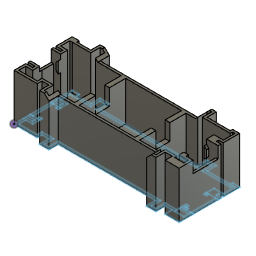
ICC Plug v2 v21 (Autodesk Fusion 360 design; units mm, degrees)
Autodesk Fusion 360 part; units mm, degrees
note: some values were not read from the file. Set by a fixed rule: which sketch regions a step uses.
sketch "Sketch1" plane through (0, 0, 0) normal (0, 1, 0) x (1, 0, 0)
  line L0 (3, 25) -> (0, 25)
  line L1 (0, 25) -> (0, 19)
  line L2 (0, 18) -> (3, 18)
  line L3 (3, 18) -> (3, 17)
  line L4 (3, 17) -> (0, 17)
  line L5 (0, 16) -> (0, 7)
  line L6 (0, 6) -> (3, 6)
  line L7 (3, 6) -> (3, 5)
  line L8 (3, 5) -> (0, 5)
  line L9 (0, 4) -> (0, 0)
  line L10 (0, 0) -> (10, 0)
  line L11 (10, 0) -> (10, 2)
  line L12 (10, 2) -> (13, 2)
  line L13 (13, 2) -> (13, -2)
  line L14 (13, -2) -> (17, -2)
  line L15 (17, -2) -> (17, 2)
  line L16 (17, 2) -> (59, 2)
  line L17 (59, 2) -> (59, -2)
  line L18 (59, -2) -> (63, -2)
  line L19 (63, -2) -> (63, 2)
  line L20 (63, 2) -> (66, 2)
  line L21 (66, 2) -> (66, -1.0002)
  line L22 (66, -1.0002) -> (72, -1.0002)
  line L23 (72, 24.9998) -> (69, 24.9998)
  line L24 (69, 24.9998) -> (69, 23.9998)
  line L25 (69, 23.9998) -> (59, 23.9998)
  line L26 (59, 23.9998) -> (59, 27.9998)
  line L27 (59, 27.9998) -> (55, 27.9998)
  line L28 (55, 27.9998) -> (55, 23.9998)
  line L29 (55, 23.9998) -> (13, 24)
  line L30 (13, 24) -> (13, 28)
  line L31 (13, 28) -> (9, 28)
  line L32 (9, 28) -> (9, 24)
  line L33 (9, 24) -> (3, 24)
  line L34 (3, 25) -> (3, 24)
  line L35 (72, -1.0002) -> (72, 4.9998)
  line L36 (72, 16.9998) -> (70, 16.9998)
  line L37 (70, 16.9998) -> (70, 17.9998)
  line L38 (70, 17.9998) -> (72, 17.9998)
  line L39 (72, 24.9998) -> (72, 18.9998)
  line L40 (72, 16.9998) -> (72, 15.7629)
  line L41 (72, 17.9998) -> (72, 18.9998)
  line L42 (0, 18) -> (0, 19)
  line L43 (0, 17) -> (0, 16)
  line L44 (0, 6) -> (0, 7)
  line L45 (0, 5) -> (0, 4)
  line L46 (12, 27) -> (10, 27)
  line L47 (10, 27) -> (10, 23)
  line L48 (10, 23) -> (2, 23)
  line L49 (1, 23) -> (1, 19)
  line L50 (1, 19) -> (4, 19)
  line L51 (4, 19) -> (4, 16)
  line L52 (4, 16) -> (1, 16)
  line L53 (1, 16) -> (1, 7)
  line L54 (1, 7) -> (4, 7)
  line L55 (4, 7) -> (4, 4)
  line L56 (4, 4) -> (1, 4)
  line L57 (1, 4) -> (1, 1)
  line L58 (1, 1) -> (9, 1)
  line L59 (9, 1) -> (9, 3)
  line L60 (9, 3) -> (14, 3)
  line L61 (14, 3) -> (14, -1)
  line L62 (14, -1) -> (16, -1)
  line L63 (16, -1) -> (16, 3)
  line L64 (16, 3) -> (60, 3)
  line L65 (60, 3) -> (60, -1)
  line L66 (60, -1) -> (62, -1)
  line L67 (62, -1) -> (62, 3)
  line L68 (62, 3) -> (67, 3)
  line L69 (67, 3) -> (67, 1.9998)
  line L70 (67, 1.9998) -> (71, 1.9998)
  line L71 (71, 1.9998) -> (71, 4.9998)
  line L72 (71, 15.7629) -> (67, 15.7629)
  line L73 (67, 15.7629) -> (67, 18.9998)
  line L74 (67, 18.9998) -> (71, 18.9998)
  line L75 (71, 23.9998) -> (71, 18.9998)
  line L76 (71, 23.9998) -> (70, 23.9998)
  line L77 (70, 23.9998) -> (70, 22.9998)
  line L78 (70, 22.9998) -> (58, 22.9998)
  line L79 (58, 22.9998) -> (58, 26.9998)
  line L80 (58, 26.9998) -> (56, 26.9998)
  line L81 (56, 26.9998) -> (56, 22.9998)
  line L82 (56, 22.9998) -> (12, 23)
  line L83 (12, 23) -> (12, 27)
  line L84 (72, 4.9998) -> (71, 4.9998)
  line L85 (71, 4.9998) -> (69, 4.9998)
  line L86 (69, 4.9998) -> (69, 5.9998)
  line L87 (69, 5.9998) -> (68, 5.9998)
  line L88 (72, 15.7629) -> (71, 15.7629)
  line L89 (71, 15.7629) -> (71, 4.9998)
  line L90 (72, 4.9998) -> (72, 15.7629)
  line L91 (68, 5.9998) -> (68, 6.9998)
  line L92 (68, 6.9998) -> (67, 6.9998)
  line L93 (67, 6.9998) -> (67, 4)
  line L94 (67, 4) -> (71, 4)
  line L95 (67, 15.7629) -> (67, 14.7629)
  line L96 (67, 14.7629) -> (68, 14.7629)
  line L97 (68, 14.7629) -> (68, 15.7629)
  line L98 (68, 5.9998) -> (67, 5.9998)
  line L99 (69, 4.9998) -> (67, 4.9998)
  line L100 (1, 7) -> (0, 7)
  line L101 (1, 16) -> (0, 16)
  line L102 (4, 16) -> (4, 15)
  line L103 (4, 15) -> (3, 15)
  line L104 (3, 15) -> (3, 16)
  line L105 (4, 7) -> (4, 8)
  line L106 (4, 8) -> (3, 8)
  line L107 (3, 8) -> (3, 7)
  line L108 (68, 5.9998) -> (68, 4.9998)
  line L109 (2, 23) -> (1, 23)
  dimension "d10" = 7
  dimension "d11" = 3
  dimension "d12" = 1
  dimension "d13" = 3
  dimension "d14" = 11
  dimension "d15" = 3
  dimension "d16" = 1
  dimension "d17" = 3
  dimension "d18" = 5
  dimension "d47" = 1
  dimension "d48" = 3
  dimension "d49" = 6
  dimension "d50" = 4
  dimension "d51" = 4
  dimension "d52" = 4
  dimension "d53" = 42
  dimension "d54" = 4
  dimension "d55" = 4
  dimension "d56" = 4
  dimension "d57" = 10
  dimension "d58" = 3
  dimension "d59" = 1
  dimension "d60" = 7
  dimension "d62" = 1
  dimension "d64" = 18
  dimension "d65" = 6
  dimension "d66" = 3
  dimension "d67" = 4
  dimension "d68" = 4
  dimension "d69" = 4
  dimension "d70" = 42
  dimension "d71" = 4
  dimension "d72" = 4
  dimension "d73" = 4
  dimension "d74" = 3
  dimension "d75" = 10
  dimension "d76" = 2
  dimension "d77" = 2
  dimension "d93" = 6
  dimension "d94" = 2
  dimension "d97" = 1
  dimension "d98" = 1
  dimension "d99" = 1
  dimension "d100" = 1
  dimension "d102" = 4
  dimension "d103" = 1
  dimension "d104" = 1
  dimension "d105" = 1
  dimension "d106" = 1
  dimension "d107" = 1
  dimension "d108" = 1
  dimension "d142" = 2
  constraint perpendicular L0 L1
  constraint perpendicular L2 L3
  constraint perpendicular L3 L4
  constraint perpendicular L4 L5
  constraint perpendicular L5 L6
  constraint perpendicular L6 L7
  constraint perpendicular L7 L8
  constraint perpendicular L8 L9
  constraint perpendicular L9 L10
  constraint perpendicular L10 L11
  constraint perpendicular L11 L12
  constraint perpendicular L12 L13
  constraint perpendicular L13 L14
  constraint perpendicular L14 L15
  constraint perpendicular L15 L16
  constraint perpendicular L14 L17
  constraint perpendicular L17 L18
  constraint perpendicular L18 L19
  constraint perpendicular L19 L20
  constraint perpendicular L20 L21
  constraint perpendicular L19 L22
  constraint perpendicular L23 L24
  constraint perpendicular L24 L25
  constraint perpendicular L25 L26
  constraint perpendicular L26 L27
  constraint perpendicular L27 L28
  constraint perpendicular L28 L29
  constraint perpendicular L25 L30
  constraint perpendicular L30 L31
  constraint perpendicular L31 L32
  constraint perpendicular L32 L33
  constraint perpendicular L33 L34
  constraint perpendicular L22 L35
  constraint perpendicular L35 L36
  constraint perpendicular L36 L37
  constraint perpendicular L35 L38
  constraint perpendicular L38 L39
  constraint coincident L9.end L10.start
  constraint perpendicular L36 L40
  constraint perpendicular L38 L41
  constraint perpendicular L4 L43
  constraint perpendicular L71 L84
  constraint parallel L31 L46
  constraint parallel L32 L47
  constraint parallel L33 L48
  constraint parallel L1 L49
  constraint parallel L2 L50
  constraint parallel L3 L51
  constraint parallel L4 L52
  constraint parallel L5 L53
  constraint parallel L6 L54
  constraint parallel L7 L55
  constraint parallel L8 L56
  constraint parallel L9 L57
  constraint parallel L10 L58
  constraint parallel L11 L59
  constraint parallel L12 L60
  constraint parallel L13 L61
  constraint parallel L14 L62
  constraint parallel L15 L63
  constraint parallel L16 L64
  constraint parallel L17 L65
  constraint parallel L18 L66
  constraint parallel L19 L67
  constraint parallel L20 L68
  constraint parallel L21 L69
  constraint parallel L22 L70
  constraint parallel L35 L71
  constraint parallel L36 L72
  constraint parallel L37 L73
  constraint parallel L38 L74
  constraint parallel L39 L75
  constraint parallel L23 L76
  constraint parallel L24 L77
  constraint parallel L25 L78
  constraint parallel L26 L79
  constraint parallel L27 L80
  constraint parallel L28 L81
  constraint parallel L29 L82
  constraint parallel L30 L83
  constraint perpendicular L71 L85
  constraint perpendicular L85 L86
  constraint perpendicular L86 L87
  constraint perpendicular L40 L88
  constraint perpendicular L85 L89
  constraint perpendicular L88 L90
  constraint perpendicular L87 L91
  constraint perpendicular L91 L92
  constraint perpendicular L92 L93
  constraint coincident L71 L94.end
  constraint perpendicular L71 L94
  constraint perpendicular L72 L95
  constraint perpendicular L73 L96
  constraint coincident L72 L97.end
  constraint perpendicular L72 L97
  constraint coincident L93 L98.end
  constraint perpendicular L93 L98
  constraint coincident L93 L99.end
  constraint perpendicular L93 L99
  constraint perpendicular L5 L100
  constraint perpendicular L5 L101
  constraint perpendicular L52 L102
  constraint perpendicular L102 L103
  constraint coincident L52 L104.end
  constraint perpendicular L52 L104
  constraint perpendicular L54 L105
  constraint perpendicular L105 L106
  constraint coincident L54 L107.end
  constraint perpendicular L54 L107
  constraint midpoint L99 L108.end
  constraint perpendicular L49 L109
  measures "d10" distance of L0.end L2.start
  measures "d11" distance of L2.start L2.end
  measures "d12" distance of L2.end L3.end L13
  measures "d13" distance of L3.end L4.end L13
  measures "d14" distance of L4.end L6.start
  measures "d15" distance of L6.start L6.end
  measures "d16" distance of L6.end L7.end
  measures "d17" distance of L7.end L8.end
  measures "d18" distance of L8.end L9.end
  measures "d47" distance of L0.start L33.end L13
  measures "d48" distance of L0.start L0.end L13
  measures "d49" distance of L32.end L33.end
  measures "d50" distance of L31.end L32.end
  measures "d51" distance of L29.end L30.end L13
  measures "d52" distance of L30.end L31.end L13
  measures "d53" distance of L28.end L29.end
  measures "d54" distance of L27.end L28.end
  measures "d55" distance of L25.end L26.end
  measures "d56" distance of L26.end L27.end
  measures "d57" horizontal distance of L24.end L25.end
  measures "d58" distance of L23.start L23.end
  measures "d59" distance of L23.end L24.end
  measures "d60" distance of L23.start L38.end
  measures "d62" distance of L36.end L37.end
  measures "d64" distance of L22.end L36.start
  measures "d65" distance of L21.end L22.end
  measures "d66" distance of L19.end L20.end
  measures "d67" distance of L18.end L19.end
  measures "d68" distance of L17.end L18.end
  measures "d69" distance of L16.end L17.end
  measures "d70" distance of L15.end L16.end
  measures "d71" distance of L14.end L15.end
  measures "d72" distance of L13.end L14.end
  measures "d73" distance of L12.end L13.end L76.end
  measures "d74" distance of L11.end L12.end
  measures "d75" distance of L9.end L10.end
  measures "d76" distance of L37.end L38.end
  measures "d77" distance of L36.start L36.end
  measures "d93" distance of L22 L84
  measures "d94" distance of L71.end L85.end
  measures "d97" distance of L85.end L86.end
  measures "d98" distance of L86.end L87.end
  measures "d99" distance of L91.end L92.end
  measures "d100" distance of L87.end L91.end
  measures "d102" distance of L72.start L72.end
  measures "d103" distance of L72.end L95.end
  measures "d104" distance of L95.end L96.end
  measures "d105" distance of L51.end L102.end
  measures "d106" distance of L102.end L103.end
  measures "d107" distance of L54.end L105.end
  measures "d108" distance of L105.end L106.end
  measures "d142" distance of L58.end L59.end
extrude "Extrude3" add sketch "Sketch1" along normal blind 20 contours L0 L1 L2 L3 L4 L23 L24 L25 L26 L27 L28 L29 L30 L31 L32 L33 L34 L36 L37 L38 L39 L40 L41 L42 L43 L46 L47 L48 L49 L50 L51 L52 L72 L73 L74 L75 L76 L77 L78 L79 L80 L81 L82 L83 L88 L101 L109 | L6 L7 L8 L9 L10 L11 L12 L13 L14 L15 L16 L17 L18 L19 L20 L21 L22 L35 L44 L45 L54 L55 L56 L57 L58 L59 L60 L61 L62 L63 L64 L65 L66 L67 L68 L69 L70 L71 L84 L100 | L71 L85 L93 L94 L99 | L86 L87 L99 L108 | L93 L98 L99 L108 makes body 1 at (41.3333, 6.6667, -22.9999) makes body 2 at (30.6667, 6.6667, -3)
extrude "Extrude4" add sketch "Sketch1" along normal blind 15 contours L5 L53 L100 L101 | L84 L88 L89 L90 bodies 1 2
extrude "Extrude5" add sketch "Sketch1" along normal blind 18 contours L52 L102 L103 L104 | L54 L105 L106 L107 | L72 L95 L96 L97 | L91 L92 L93 L98 bodies 1
extrude "Extrude6" cut sketch "Sketch1" along normal blind 13 contours L52 L102 L103 L104 | L54 L105 L106 L107 | L72 L95 L96 L97 | L91 L92 L93 L98 bodies 1
sketch "Sketch3" plane through (0.0001, 0, -28) normal (0.000003, 0, -1) x (-1, 0, -0.000003)
  line L0 (-12.9999, 0) -> (-8.9999, 0)
  line L1 (-8.9999, 0) -> (-8.9999, 20)
  line L2 (-8.9999, 20) -> (-12.9999, 20)
  line L3 (-12.9999, 20) -> (-12.9999, 0)
  line L4 (-10.9999, 20) -> (-12.9999, 18)
  line L5 (-10.9999, 20) -> (-13.8284, 20) construction
  line L6 (-12.9999, 18) -> (-55, 18)
  line L7 (-55, 18) -> (-57, 20)
  line L8 (-57, 20) -> (-10.9999, 20)
  dimension "d131" = 45
  constraint horizontal L5
  constraint midpoint L2 L4.start
  constraint coincident L3 L4.end
  constraint perpendicular L3 L6
  measures "d131" angle of L4 L5
extrude "Extrude9" cut sketch "Sketch3" against normal up to surface (5 mm away) contours L3 L6 L7 L8 | L2 L3 L4 L8 bodies 1
sketch "Sketch4" plane through (0, 0, 2) normal (0, 0, 1) x (1, 0, 0)
  line L0 (13, 0) -> (17, 0)
  line L1 (17, 0) -> (17, 20)
  line L2 (17, 20) -> (13, 20)
  line L3 (13, 20) -> (13, 0)
  line L4 (15, 20) -> (17, 18)
  line L5 (15, 20) -> (17.8284, 20) construction
  line L6 (17, 18) -> (59, 18)
  line L7 (59, 18) -> (61, 20)
  line L8 (61, 20) -> (15, 20)
  dimension "d134" = 45
  constraint horizontal L5
  constraint midpoint L2 L4.start
  constraint coincident L1 L4.end
  constraint perpendicular L1 L6
  measures "d134" angle of L4 L5
extrude "Extrude10" cut sketch "Sketch4" against normal up to surface (5 mm away) contours L1 L2 L4 L8 | L1 L6 L7 L8 bodies 1
chamfer "Chamfer2" distance 1 angle 45 8 edges at (68, 18, -15.2629) (68, 13, -15.2629) (68, 18, -6.4998) (68, 13, -6.4998) (3, 13, -15.5) (3, 18, -15.5) (3, 18, -7.5) (3, 13, -7.5) on bodies 1
extrude "Extrude11" add sketch "Sketch1" along normal blind 1 contours L46 L47 L48 L49 L50 L51 L52 L53 L54 L55 L56 L57 L58 L59 L60 L61 L62 L63 L64 L65 L66 L67 L68 L69 L70 L71 L72 L73 L74 L75 L76 L77 L78 L79 L80 L81 L82 L83 L85 L86 L87 L89 L91 L92 L93 L94 L95 L96 L97 L102 L103 L104 L105 L106 L107 L109 | L52 L102 L103 L104 | L54 L105 L106 L107 | L72 L95 L96 L97 | L91 L92 L93 L98 bodies 1
sketch "Sketch5" plane through (0, 0, 0) normal (0, 1, 0) x (1, 0, 0)
  line L0 (4, 8) -> (4, 15)
  line L1 (4, 15) -> (1, 15)
  line L2 (1, 15) -> (1, 8)
  line L3 (1, 8) -> (4, 8)
  line L4 (67, 7) -> (67, 14.7555)
  line L5 (67, 14.7555) -> (71, 14.7555)
  line L6 (71, 14.7555) -> (71, 7)
  line L7 (71, 7) -> (67, 7)
  constraint vertical L0
  constraint perpendicular L0 L1
  constraint perpendicular L1 L2
  constraint perpendicular L0 L3
  constraint perpendicular L3 L4
  constraint perpendicular L4 L5
  constraint perpendicular L5 L6
  constraint perpendicular L6 L7
extrude "Extrude12" cut sketch "Sketch5" along normal up to surface (1 mm away) bodies 1
sketch "Sketch6" plane through (0, 1, 0) normal (0, 1, 0) x (-1, 0, 0)
  line L0 (-4, -8) -> (-1, -8)
  line L1 (-1, -8) -> (-1, -7)
  line L2 (-1, -7) -> (-4, -7)
  line L3 (-4, -7) -> (-4, -4)
  line L4 (-4, -4) -> (-1, -4)
  line L5 (-1, -4) -> (-1, -1)
  line L6 (-1, -1) -> (-9, -1)
  line L7 (-9, -1) -> (-9, -3)
  line L8 (-9, -3) -> (-14, -3)
  line L9 (-14, -3) -> (-14, 1)
  line L10 (-14, 1) -> (-16, 1)
  line L11 (-16, 1) -> (-16, -3)
  line L12 (-16, -3) -> (-60, -3)
  line L13 (-60, -3) -> (-60, 1)
  line L14 (-60, 1) -> (-62, 1)
  line L15 (-62, 1) -> (-62, -3)
  line L16 (-62, -3) -> (-67, -3)
  line L17 (-67, -3) -> (-67, -1.9998)
  line L18 (-67, -1.9998) -> (-71, -1.9998)
  line L19 (-71, -1.9998) -> (-71, -4)
  line L20 (-71, -4) -> (-67, -4)
  line L21 (-67, -4) -> (-67, -5.9998)
  line L22 (-67, -5.9998) -> (-69, -5.9998)
  line L23 (-69, -5.9998) -> (-69, -4.9998)
  line L24 (-69, -4.9998) -> (-71, -4.9998)
  line L25 (-71, -4.9998) -> (-71, -7)
  line L26 (-71, -7) -> (-67, -7)
  line L27 (-67, -7) -> (-67, -14.7555)
  line L28 (-67, -14.7555) -> (-71, -14.7555)
  line L29 (-71, -14.7555) -> (-71, -15.7629)
  line L30 (-71, -15.7629) -> (-67, -15.7629)
  line L31 (-67, -15.7629) -> (-67, -18.9998)
  line L32 (-67, -18.9998) -> (-71, -18.9998)
  line L33 (-71, -18.9998) -> (-71, -23.9998)
  line L34 (-71, -23.9998) -> (-70, -23.9998)
  line L35 (-70, -23.9998) -> (-70, -22.9998)
  line L36 (-70, -22.9998) -> (-58, -22.9998)
  line L37 (-58, -22.9998) -> (-58, -26.9998)
  line L38 (-58, -26.9998) -> (-56, -26.9998)
  line L39 (-56, -26.9998) -> (-56, -22.9998)
  line L40 (-56, -22.9998) -> (-12, -23)
  line L41 (-12, -23) -> (-12, -27)
  line L42 (-12, -27) -> (-10, -27)
  line L43 (-10, -27) -> (-10, -23)
  line L44 (-10, -23) -> (-2, -23)
  line L45 (-2, -23) -> (-1, -23)
  line L46 (-1, -23) -> (-1, -19)
  line L47 (-1, -19) -> (-4, -19)
  line L48 (-4, -19) -> (-4, -16)
  line L49 (-4, -16) -> (-1, -16)
  line L50 (-1, -16) -> (-1, -15)
  line L51 (-1, -15) -> (-4, -15)
  line L52 (-4, -15) -> (-4, -8)
  line L53 (-23, -22.9999) -> (-25, -22.9999)
  line L54 (-25, -22.9999) -> (-25, -2.9999)
  line L55 (-25, -2.9999) -> (-23, -2.9999)
  line L56 (-23, -2.9999) -> (-23, -22.9999)
  line L57 (-4, -19) -> (-4, -16)
  line L58 (-49, -22.9999) -> (-51, -22.9999)
  line L59 (-51, -22.9999) -> (-51, -2.9999)
  line L60 (-51, -2.9999) -> (-49, -2.9999)
  line L61 (-49, -2.9999) -> (-49, -22.9999)
  line L62 (-67, -15.7629) -> (-67, -18.9998)
  line L63 (-23, -15.9999) -> (-25, -15.9999)
  line L64 (-25, -15.9999) -> (-25, -9.9999)
  line L65 (-25, -9.9999) -> (-23, -9.9999)
  line L66 (-23, -9.9999) -> (-23, -15.9999)
  line L67 (-49, -15.9999) -> (-51, -15.9999)
  line L68 (-51, -15.9999) -> (-51, -9.9999)
  line L69 (-51, -9.9999) -> (-49, -9.9999)
  line L70 (-49, -9.9999) -> (-49, -15.9999)
  dimension "d143" = 2
  dimension "d144" = 20
  dimension "d145" = 19
  dimension "d146" = 2
  dimension "d147" = 20
  dimension "d148" = 16
  dimension "d149" = 2
  dimension "d150" = 6
  dimension "d151" = 7
  dimension "d152" = 2
  dimension "d153" = 6
  dimension "d154" = 7
  constraint horizontal L53
  constraint vertical L54
  constraint horizontal L55
  constraint vertical L56
  constraint coincident L40 L53.start
  constraint horizontal L58
  constraint vertical L59
  constraint horizontal L60
  constraint vertical L61
  constraint coincident L40 L58.start
  constraint horizontal L63
  constraint vertical L64
  constraint horizontal L65
  constraint vertical L66
  constraint coincident L56 L63.start
  constraint horizontal L67
  constraint vertical L68
  constraint horizontal L69
  constraint vertical L70
  constraint coincident L61 L67.start
  measures "d143" distance of L53.start L53.end
  measures "d144" distance of L53.start L55.end
  measures "d145" distance of L56 L57
  measures "d146" distance of L58.start L58.end
  measures "d147" distance of L58.start L60.end
  measures "d148" distance of L59 L62
  measures "d149" distance of L63.start L63.end
  measures "d150" distance of L63.start L65.end
  measures "d151" distance of L53 L63
  measures "d152" distance of L67.start L67.end
  measures "d153" distance of L67.start L69.end
  measures "d154" distance of L58 L67
extrude "Extrude13" add sketch "Sketch6" along normal up to surface (17 mm away) contours L12 L54 L55 L56 L65 | L40 L53 L54 L56 L63 | L12 L59 L60 L61 L69 | L40 L58 L59 L61 L67 bodies 1
extrude "Extrude14" add sketch "Sketch6" along normal blind 10 contours L54 L56 L63 L64 L65 L66 | L59 L61 L67 L68 L69 L70 bodies 1
sketch "Sketch7" plane through (0, 1, 0) normal (0, 1, 0) x (-1, 0, 0)
  line L0 (-23, -3) -> (-23, -22.9999)
  line L1 (-23, -22.9999) -> (-12, -23)
  line L2 (-12, -23) -> (-12, -27)
  line L3 (-12, -27) -> (-10, -27)
  line L4 (-10, -27) -> (-10, -23)
  line L5 (-10, -23) -> (-2, -23)
  line L6 (-2, -23) -> (-1, -23)
  line L7 (-1, -23) -> (-1, -19)
  line L8 (-1, -19) -> (-4, -19)
  line L9 (-4, -19) -> (-4, -16)
  line L10 (-4, -16) -> (-1, -16)
  line L11 (-1, -16) -> (-1, -15)
  line L12 (-1, -15) -> (-4, -15)
  line L13 (-4, -15) -> (-4, -8)
  line L14 (-4, -8) -> (-1, -8)
  line L15 (-1, -8) -> (-1, -7)
  line L16 (-1, -7) -> (-4, -7)
  line L17 (-4, -7) -> (-4, -4)
  line L18 (-4, -4) -> (-1, -4)
  line L19 (-1, -4) -> (-1, -1)
  line L20 (-1, -1) -> (-9, -1)
  line L21 (-9, -1) -> (-9, -3)
  line L22 (-9, -3) -> (-14, -3)
  line L23 (-14, -3) -> (-14, 1)
  line L24 (-14, 1) -> (-16, 1)
  line L25 (-16, 1) -> (-16, -3)
  line L26 (-16, -3) -> (-23, -3)
  line L27 (-6.5, -18) -> (-9, -18)
  line L28 (-9, -18) -> (-9, -17)
  line L29 (-9, -17) -> (-6.5, -17)
  line L30 (-6.5, -17) -> (-6.5, -18)
  line L31 (-10, -23) -> (-2, -23)
  line L32 (-4, -19) -> (-4, -16)
  line L33 (-27, -17.9999) -> (-28.5, -17.9999)
  line L34 (-28.5, -17.9999) -> (-28.5, -16.9999)
  line L35 (-28.5, -16.9999) -> (-27, -16.9999)
  line L36 (-27, -16.9999) -> (-27, -17.9999)
  line L37 (-56, -22.9998) -> (-12, -23)
  line L38 (-25, -22.9999) -> (-25, -15.9999)
  line L39 (-10.5, -17) -> (-10.5, -18)
  line L40 (-10.5, -18) -> (-13, -18)
  line L41 (-13, -17) -> (-10.5, -17)
  line L42 (-13, -18) -> (-13, -17)
  line L43 (-14.5, -17) -> (-14.5, -18)
  line L44 (-14.5, -18) -> (-17, -18)
  line L45 (-17, -17) -> (-14.5, -17)
  line L46 (-17, -18) -> (-17, -17)
  line L47 (-18.5, -17) -> (-18.5, -18)
  line L48 (-18.5, -18) -> (-21, -18)
  line L49 (-21, -17) -> (-18.5, -17)
  line L50 (-21, -18) -> (-21, -17)
  line L51 (-6.5, -12) -> (-6.5, -13)
  line L52 (-6.5, -13) -> (-9, -13)
  line L53 (-9, -12) -> (-6.5, -12)
  line L54 (-9, -13) -> (-9, -12)
  line L55 (-10.5, -12) -> (-10.5, -13)
  line L56 (-10.5, -13) -> (-13, -13)
  line L57 (-13, -12) -> (-10.5, -12)
  line L58 (-13, -13) -> (-13, -12)
  line L59 (-14.5, -12) -> (-14.5, -13)
  line L60 (-14.5, -13) -> (-17, -13)
  line L61 (-17, -12) -> (-14.5, -12)
  line L62 (-17, -13) -> (-17, -12)
  line L63 (-18.5, -12) -> (-18.5, -13)
  line L64 (-18.5, -13) -> (-21, -13)
  line L65 (-21, -12) -> (-18.5, -12)
  line L66 (-21, -13) -> (-21, -12)
  line L67 (-6.5, -7) -> (-6.5, -8)
  line L68 (-6.5, -8) -> (-9, -8)
  line L69 (-9, -7) -> (-6.5, -7)
  line L70 (-9, -8) -> (-9, -7)
  line L71 (-10.5, -7) -> (-10.5, -8)
  line L72 (-10.5, -8) -> (-13, -8)
  line L73 (-13, -7) -> (-10.5, -7)
  line L74 (-13, -8) -> (-13, -7)
  line L75 (-14.5, -7) -> (-14.5, -8)
  line L76 (-14.5, -8) -> (-17, -8)
  line L77 (-17, -7) -> (-14.5, -7)
  line L78 (-17, -8) -> (-17, -7)
  line L79 (-18.5, -7) -> (-18.5, -8)
  line L80 (-18.5, -8) -> (-21, -8)
  line L81 (-21, -7) -> (-18.5, -7)
  line L82 (-21, -8) -> (-21, -7)
  line L83 (-53, -17.9998) -> (-54.5, -17.9998)
  line L84 (-54.5, -17.9998) -> (-54.5, -16.9998)
  line L85 (-54.5, -16.9998) -> (-53, -16.9998)
  line L86 (-53, -16.9998) -> (-53, -17.9998)
  line L87 (-51, -22.9999) -> (-51, -15.9999)
  line L88 (-31.0714, -17.9999) -> (-31.0714, -16.9999)
  line L89 (-31.0714, -16.9999) -> (-29.5714, -16.9999)
  line L90 (-29.5714, -16.9999) -> (-29.5714, -17.9999)
  line L91 (-29.5714, -17.9999) -> (-31.0714, -17.9999)
  line L92 (-33.6429, -17.9999) -> (-33.6429, -16.9999)
  line L93 (-33.6429, -16.9999) -> (-32.1429, -16.9999)
  line L94 (-32.1429, -16.9999) -> (-32.1429, -17.9999)
  line L95 (-32.1429, -17.9999) -> (-33.6429, -17.9999)
  line L96 (-36.2143, -17.9999) -> (-36.2143, -16.9999)
  line L97 (-36.2143, -16.9999) -> (-34.7143, -16.9999)
  line L98 (-34.7143, -16.9999) -> (-34.7143, -17.9999)
  line L99 (-34.7143, -17.9999) -> (-36.2143, -17.9999)
  line L100 (-38.7857, -17.9999) -> (-38.7857, -16.9999)
  line L101 (-38.7857, -16.9999) -> (-37.2857, -16.9999)
  line L102 (-37.2857, -16.9999) -> (-37.2857, -17.9999)
  line L103 (-37.2857, -17.9999) -> (-38.7857, -17.9999)
  line L104 (-41.3571, -17.9999) -> (-41.3571, -16.9999)
  line L105 (-41.3571, -16.9999) -> (-39.8571, -16.9999)
  line L106 (-39.8571, -16.9999) -> (-39.8571, -17.9999)
  line L107 (-39.8571, -17.9999) -> (-41.3571, -17.9999)
  line L108 (-43.9286, -17.9999) -> (-43.9286, -16.9999)
  line L109 (-43.9286, -16.9999) -> (-42.4286, -16.9999)
  line L110 (-42.4286, -16.9999) -> (-42.4286, -17.9999)
  line L111 (-42.4286, -17.9999) -> (-43.9286, -17.9999)
  line L112 (-46.5, -17.9999) -> (-46.5, -16.9999)
  line L113 (-46.5, -16.9999) -> (-45, -16.9999)
  line L114 (-45, -16.9999) -> (-45, -17.9999)
  line L115 (-45, -17.9999) -> (-46.5, -17.9999)
  line L116 (-28.5, -12.9999) -> (-28.5, -11.9999)
  line L117 (-28.5, -11.9999) -> (-27, -11.9999)
  line L118 (-27, -11.9999) -> (-27, -12.9999)
  line L119 (-27, -12.9999) -> (-28.5, -12.9999)
  line L120 (-31.0714, -12.9999) -> (-31.0714, -11.9999)
  line L121 (-31.0714, -11.9999) -> (-29.5714, -11.9999)
  line L122 (-29.5714, -11.9999) -> (-29.5714, -12.9999)
  line L123 (-29.5714, -12.9999) -> (-31.0714, -12.9999)
  line L124 (-33.6429, -12.9999) -> (-33.6429, -11.9999)
  line L125 (-33.6429, -11.9999) -> (-32.1429, -11.9999)
  line L126 (-32.1429, -11.9999) -> (-32.1429, -12.9999)
  line L127 (-32.1429, -12.9999) -> (-33.6429, -12.9999)
  line L128 (-36.2143, -12.9999) -> (-36.2143, -11.9999)
  line L129 (-36.2143, -11.9999) -> (-34.7143, -11.9999)
  line L130 (-34.7143, -11.9999) -> (-34.7143, -12.9999)
  line L131 (-34.7143, -12.9999) -> (-36.2143, -12.9999)
  line L132 (-38.7857, -12.9999) -> (-38.7857, -11.9999)
  line L133 (-38.7857, -11.9999) -> (-37.2857, -11.9999)
  line L134 (-37.2857, -11.9999) -> (-37.2857, -12.9999)
  line L135 (-37.2857, -12.9999) -> (-38.7857, -12.9999)
  line L136 (-41.3571, -12.9999) -> (-41.3571, -11.9999)
  line L137 (-41.3571, -11.9999) -> (-39.8571, -11.9999)
  line L138 (-39.8571, -11.9999) -> (-39.8571, -12.9999)
  line L139 (-39.8571, -12.9999) -> (-41.3571, -12.9999)
  line L140 (-43.9286, -12.9999) -> (-43.9286, -11.9999)
  line L141 (-43.9286, -11.9999) -> (-42.4286, -11.9999)
  line L142 (-42.4286, -11.9999) -> (-42.4286, -12.9999)
  line L143 (-42.4286, -12.9999) -> (-43.9286, -12.9999)
  line L144 (-46.5, -12.9999) -> (-46.5, -11.9999)
  line L145 (-46.5, -11.9999) -> (-45, -11.9999)
  line L146 (-45, -11.9999) -> (-45, -12.9999)
  line L147 (-45, -12.9999) -> (-46.5, -12.9999)
  line L148 (-28.5, -7.9999) -> (-28.5, -6.9999)
  line L149 (-28.5, -6.9999) -> (-27, -6.9999)
  line L150 (-27, -6.9999) -> (-27, -7.9999)
  line L151 (-27, -7.9999) -> (-28.5, -7.9999)
  line L152 (-31.0714, -7.9999) -> (-31.0714, -6.9999)
  line L153 (-31.0714, -6.9999) -> (-29.5714, -6.9999)
  line L154 (-29.5714, -6.9999) -> (-29.5714, -7.9999)
  line L155 (-29.5714, -7.9999) -> (-31.0714, -7.9999)
  line L156 (-33.6429, -7.9999) -> (-33.6429, -6.9999)
  line L157 (-33.6429, -6.9999) -> (-32.1429, -6.9999)
  line L158 (-32.1429, -6.9999) -> (-32.1429, -7.9999)
  line L159 (-32.1429, -7.9999) -> (-33.6429, -7.9999)
  line L160 (-36.2143, -7.9999) -> (-36.2143, -6.9999)
  line L161 (-36.2143, -6.9999) -> (-34.7143, -6.9999)
  line L162 (-34.7143, -6.9999) -> (-34.7143, -7.9999)
  line L163 (-34.7143, -7.9999) -> (-36.2143, -7.9999)
  line L164 (-38.7857, -7.9999) -> (-38.7857, -6.9999)
  line L165 (-38.7857, -6.9999) -> (-37.2857, -6.9999)
  line L166 (-37.2857, -6.9999) -> (-37.2857, -7.9999)
  line L167 (-37.2857, -7.9999) -> (-38.7857, -7.9999)
  line L168 (-41.3571, -7.9999) -> (-41.3571, -6.9999)
  line L169 (-41.3571, -6.9999) -> (-39.8571, -6.9999)
  line L170 (-39.8571, -6.9999) -> (-39.8571, -7.9999)
  line L171 (-39.8571, -7.9999) -> (-41.3571, -7.9999)
  line L172 (-43.9286, -7.9999) -> (-43.9286, -6.9999)
  line L173 (-43.9286, -6.9999) -> (-42.4286, -6.9999)
  line L174 (-42.4286, -6.9999) -> (-42.4286, -7.9999)
  line L175 (-42.4286, -7.9999) -> (-43.9286, -7.9999)
  line L176 (-46.5, -7.9999) -> (-46.5, -6.9999)
  line L177 (-46.5, -6.9999) -> (-45, -6.9999)
  line L178 (-45, -6.9999) -> (-45, -7.9999)
  line L179 (-45, -7.9999) -> (-46.5, -7.9999)
  line L180 (-55.75, -16.9998) -> (-55.75, -17.9998)
  line L181 (-57.25, -16.9998) -> (-55.75, -16.9998)
  line L182 (-55.75, -17.9998) -> (-57.25, -17.9998)
  line L183 (-57.25, -17.9998) -> (-57.25, -16.9998)
  line L184 (-58.5, -16.9998) -> (-58.5, -17.9998)
  line L185 (-60, -16.9998) -> (-58.5, -16.9998)
  line L186 (-58.5, -17.9998) -> (-60, -17.9998)
  line L187 (-60, -17.9998) -> (-60, -16.9998)
  line L188 (-61.25, -16.9998) -> (-61.25, -17.9998)
  line L189 (-62.75, -16.9998) -> (-61.25, -16.9998)
  line L190 (-61.25, -17.9998) -> (-62.75, -17.9998)
  line L191 (-62.75, -17.9998) -> (-62.75, -16.9998)
  line L192 (-64, -16.9998) -> (-64, -17.9998)
  line L193 (-65.5, -16.9998) -> (-64, -16.9998)
  line L194 (-64, -17.9998) -> (-65.5, -17.9998)
  line L195 (-65.5, -17.9998) -> (-65.5, -16.9998)
  line L196 (-53, -11.9998) -> (-53, -12.9998)
  line L197 (-54.5, -11.9998) -> (-53, -11.9998)
  line L198 (-53, -12.9998) -> (-54.5, -12.9998)
  line L199 (-54.5, -12.9998) -> (-54.5, -11.9998)
  line L200 (-55.75, -11.9998) -> (-55.75, -12.9998)
  line L201 (-57.25, -11.9998) -> (-55.75, -11.9998)
  line L202 (-55.75, -12.9998) -> (-57.25, -12.9998)
  line L203 (-57.25, -12.9998) -> (-57.25, -11.9998)
  line L204 (-58.5, -11.9998) -> (-58.5, -12.9998)
  line L205 (-60, -11.9998) -> (-58.5, -11.9998)
  line L206 (-58.5, -12.9998) -> (-60, -12.9998)
  line L207 (-60, -12.9998) -> (-60, -11.9998)
  line L208 (-61.25, -11.9998) -> (-61.25, -12.9998)
  line L209 (-62.75, -11.9998) -> (-61.25, -11.9998)
  line L210 (-61.25, -12.9998) -> (-62.75, -12.9998)
  line L211 (-62.75, -12.9998) -> (-62.75, -11.9998)
  line L212 (-64, -11.9998) -> (-64, -12.9998)
  line L213 (-65.5, -11.9998) -> (-64, -11.9998)
  line L214 (-64, -12.9998) -> (-65.5, -12.9998)
  line L215 (-65.5, -12.9998) -> (-65.5, -11.9998)
  line L216 (-53, -6.9998) -> (-53, -7.9998)
  line L217 (-54.5, -6.9998) -> (-53, -6.9998)
  line L218 (-53, -7.9998) -> (-54.5, -7.9998)
  line L219 (-54.5, -7.9998) -> (-54.5, -6.9998)
  line L220 (-55.75, -6.9998) -> (-55.75, -7.9998)
  line L221 (-57.25, -6.9998) -> (-55.75, -6.9998)
  line L222 (-55.75, -7.9998) -> (-57.25, -7.9998)
  line L223 (-57.25, -7.9998) -> (-57.25, -6.9998)
  line L224 (-58.5, -6.9998) -> (-58.5, -7.9998)
  line L225 (-60, -6.9998) -> (-58.5, -6.9998)
  line L226 (-58.5, -7.9998) -> (-60, -7.9998)
  line L227 (-60, -7.9998) -> (-60, -6.9998)
  line L228 (-61.25, -6.9998) -> (-61.25, -7.9998)
  line L229 (-62.75, -6.9998) -> (-61.25, -6.9998)
  line L230 (-61.25, -7.9998) -> (-62.75, -7.9998)
  line L231 (-62.75, -7.9998) -> (-62.75, -6.9998)
  line L232 (-64, -6.9998) -> (-64, -7.9998)
  line L233 (-65.5, -6.9998) -> (-64, -6.9998)
  line L234 (-64, -7.9998) -> (-65.5, -7.9998)
  line L235 (-65.5, -7.9998) -> (-65.5, -6.9998)
  dimension "d159" = 2.5
  dimension "d160" = 1
  dimension "d161" = 5
  dimension "d162" = 2.5
  dimension "d169" = 1.5
  dimension "d170" = 1
  dimension "d171" = 5
  dimension "d172" = 2
  dimension "d179" = -12
  dimension "d180" = 10
  dimension "d181" = 1.5
  dimension "d182" = 1
  dimension "d183" = 5
  dimension "d184" = 2
  dimension "d191" = -18
  dimension "d192" = 10
  dimension "d195" = -11
  dimension "d196" = 10
  constraint horizontal L27
  constraint vertical L28
  constraint horizontal L29
  constraint vertical L30
  constraint horizontal L33
  constraint vertical L34
  constraint horizontal L35
  constraint vertical L36
  constraint horizontal L83
  constraint vertical L84
  constraint horizontal L85
  constraint vertical L86
  measures "d159" distance of L27.start L27.end
  measures "d160" distance of L27.start L29.end
  measures "d161" distance of L27.start L31
  measures "d162" distance of L27.start L32
  measures "d169" distance of L33.start L33.end
  measures "d170" distance of L33.start L35.end
  measures "d171" distance of L33.start L37
  measures "d172" distance of L33.start L38
  measures "d181" distance of L83.start L83.end
  measures "d182" distance of L83.start L85.end
  measures "d183" distance of L37 L83.start
  measures "d184" distance of L83.start L87
extrude "Extrude15" cut sketch "Sketch7" against normal up to surface (1 mm away) contours L27 L28 L29 L30 | L33 L34 L35 L36 | L39 L40 L41 L42 | L43 L44 L45 L46 | L47 L48 L49 L50 | L51 L52 L53 L54 | L55 L56 L57 L58 | L59 L60 L61 L62 | L63 L64 L65 L66 | L67 L68 L69 L70 | L71 L72 L73 L74 | L75 L76 L77 L78 | L79 L80 L81 L82 | L83 L84 L85 L86 | L88 L89 L90 L91 | L92 L93 L94 L95 | L96 L97 L98 L99 | L100 L101 L102 L103 | L104 L105 L106 L107 | L108 L109 L110 L111 | L112 L113 L114 L115 | L116 L117 L118 L119 | L120 L121 L122 L123 | L124 L125 L126 L127 | L128 L129 L130 L131 | L132 L133 L134 L135 | L136 L137 L138 L139 | L140 L141 L142 L143 | L144 L145 L146 L147 | L148 L149 L150 L151 | L152 L153 L154 L155 | L156 L157 L158 L159 | L160 L161 L162 L163 | L164 L165 L166 L167 | L168 L169 L170 L171 | L172 L173 L174 L175 | L176 L177 L178 L179 | L180 L181 L182 L183 | L184 L185 L186 L187 | L188 L189 L190 L191 | L192 L193 L194 L195 | L196 L197 L198 L199 | L200 L201 L202 L203 | L204 L205 L206 L207 | L208 L209 L210 L211 | L212 L213 L214 L215 | L216 L217 L218 L219 | L220 L221 L222 L223 | L224 L225 L226 L227 | L228 L229 L230 L231 | L232 L233 L234 L235 bodies 1
equation "width = 1 mm"
